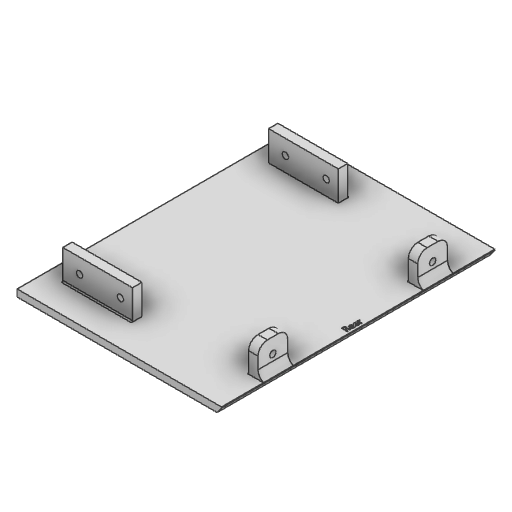
# Autodesk Inventor part: lowerSkidPlateRear
Saved by Autodesk Inventor 2025 (Build 290162000, 162)
## iProperties
Created: 2025-01-05
Part Number: lowerSkidPlateRear
Material: Generic
Document SubType Name: Modeling
Designer: derm
Density: 1 g/cm^3
Appearance: Default
Author: derm
Autodesk Inventor part; units mm, degrees
ref_plane "YZ Plane" through (0, 0, 0) normal (1, 0, 0) x (0, 1, 0)
ref_plane "XZ Plane" through (0, 0, 0) normal (0, 1, 0) x (-1, 0, 0)
ref_plane "XY Plane" through (0, 0, 0) normal (0, 0, 1) x (1, 0, 0)
sketch "Sketch1" plane through (0, 0, 0) normal (0, 1, 0) x (-1, 0, 0)
  line L0 (-87.5, 117) -> (87.5, 117)
  line L1 (87.5, 117) -> (87.5, -117)
  line L2 (87.5, -117) -> (-87.5, -117)
  line L3 (-87.5, -117) -> (-87.5, 117)
  line L4 (-87.5, 117) -> (87.5, -117) construction
  line L5 (87.5, 117) -> (-87.5, -117) construction
  point P0 (0, 0)
  dimension "d0" = 175
  dimension "d1" = 234
  constraints: 12 end point, 2 midpoint, 2 parallel, 1 horizontal, 1 perpendicular
  measures "d0" distance of L1.end L2.end
  measures "d1" distance of L0.end L1.end
extrude "Extrusion1" add sketch "Sketch1" along normal blind 6
sketch "Sketch2" plane through (0, 6, 0) normal (0, 1, 0) x (1, 0, 0)
  line L0 (87.5, 117) -> (-87.5, 117) projected
  line L1 (-87.5, 117) -> (-87.5, -117) projected
  line L2 (-87.5, -117) -> (87.5, -117) projected
  line L3 (87.5, -117) -> (87.5, 117) projected
  line L4 (76.2612, -82.1) -> (49.5135, -82.1)
  line L5 (74.806, 117.332) -> (74.806, -116.668)
  line L6 (49.5135, -82.1) -> (82.806, -82.1)
  line L7 (82.806, -82.1) -> (82.806, -55.7)
  line L8 (82.806, -55.7) -> (49.5135, -55.7)
  line L9 (49.5135, -55.7) -> (49.5135, -82.1)
  line L10 (82.806, -82.1) -> (49.5135, -82.1)
  line L11 (49.5135, -82.1) -> (49.5135, -81.1)
  line L12 (49.5135, -81.1) -> (82.806, -81.1)
  line L13 (82.806, -81.1) -> (82.806, -82.1)
  point P0 (0, 0)
  point P1 (74.806, -116.668)
  point P2 (66.1597, -55.7)
  point P3 (66.1597, -82.1)
  point P4 (74.806, -55.7)
  point P5 (70.1597, -82.1)
  point P6 (74.806, -81.1)
  dimension "d4" = 26.4
  dimension "d5" = 8
  dimension "d8" = 1
  constraints: 18 end point, 4 parallel, 2 horizontal, 2 midpoint, 2 perpendicular, 1 point on line, 3 other
  measures "d4" distance of point (66.16, -55.7) point (66.16, -82.1)
  measures "d8" distance between parallel lines of L12 L6
extrude "Extrusion2" add sketch "Sketch2" along normal blind 25.4 contours L5 L8 L7 L12
sketch "Sketch3" plane through (82.806, 6, 81.1) normal (1, 0, 0) x (0, 0, -1)
  line L0 (25.4, 0) -> (0, 0) projected
  line L1 (25.4, 0) -> (25.4, 25.4) projected
  line L2 (0, 25.4) -> (25.4, 25.4) projected
  line L3 (0, 0) -> (0, 25.4) projected
  circle A0 centre (12.7, 12.7) radius 2.75
  point P0 (81.1, -6)
  dimension "d9" = 5.5
  constraints: 1 centre point
  measures "d9" diameter of A0
extrude "Extrusion3" cut sketch "Sketch3" against normal blind 25.4 contours A0
fillet "Fillet1" radius 8 3 edges at (82.806, 6, 68.4) (78.806, 31.4, 55.7) (78.806, 31.4, 81.1)
sketch "Sketch4" plane through (0, 6, 0) normal (0, 1, 0) x (1, 0, 0)
  line L0 (87.5, -81.1) -> (74.806, -81.1) projected
  line L1 (74.806, -81.1) -> (74.806, -55.7) projected
  line L2 (74.806, -55.7) -> (87.5, -55.7) projected
  line L3 (87.5, 117) -> (-87.5, 117) projected
  line L4 (-87.5, 117) -> (-87.5, -117) projected
  line L5 (-87.5, -117) -> (87.5, -117) projected
  line L6 (87.5, -117) -> (87.5, -81.1) projected
  line L7 (-217.2403, -92.1) -> (36.7597, -92.1) projected
  line L8 (-7.3833, -87.6172) -> (32.2769, -47.957) projected
  line L9 (-13.6234, -92.1) -> (-73.3252, -92.1)
  line L10 (-73.3252, -92.1) -> (-73.3252, -84.1)
  line L11 (-73.3252, -84.1) -> (-13.6234, -84.1)
  line L12 (-13.6234, -84.1) -> (-13.6234, -92.1)
  line L13 (87.5, -55.7) -> (87.5, 117) projected
  point P0 (0, 0)
  point P1 (-73.3252, -92.1)
  dimension "d14" = 8
  constraints: 8 end point, 2 parallel, 1 horizontal, 1 perpendicular, 1 point on line, 1 vertical
  measures "d14" distance between parallel lines of L7 L11
extrude "Extrusion4" add sketch "Sketch4" along normal blind 25.4 contours L10 L11 L12 L7
sketch "Sketch5" plane through (-80, 6, 84.1) normal (0, 0, -1) x (-1, 0, 0)
  line L0 (-6.6748, 0) -> (-66.3766, 0) projected
  line L1 (-6.6748, 0) -> (-6.6748, 25.4) projected
  line L2 (-66.3766, 25.4) -> (-6.6748, 25.4) projected
  line L3 (-66.3766, 0) -> (-66.3766, 25.4) projected
  circle A0 centre (-56.0684, 12.7) radius 2.75
  circle A1 centre (-21.0684, 12.7) radius 2.75
  circle A2 centre (13.9316, 12.7) radius 2.75
  point P0 (-80, -6)
  dimension "d17" = 5.5
  dimension "d22" = 35
  constraints: 3 centre point, 1 horizontal, 4 other
  measures "d17" diameter of A0
  measures "d22" distance of A0.centre A1.centre
extrude "Extrusion5" cut sketch "Sketch5" against normal blind 25.4 contours A0 | A1 | A2
mirror "Mirror1" about plane through (0, 0, 0) normal (0, 0, 1) of "Extrusion2", "Extrusion3", "Fillet1", "Extrusion4", "Extrusion5"
sketch "Sketch8" plane through (87.5, 0, -117) normal (0, 0, -1) x (-1, 0, 0)
  line L0 (-8.2033, 16.4896) -> (-32.1539, 49.52) projected
  line L1 (0, 5.1764) -> (3.7534, 0)
  line L2 (0, 0) -> (175, 0) projected
  line L3 (175, 0) -> (175, 6) projected
  line L4 (0, 6) -> (175, 6) projected
  line L5 (0, 0) -> (0, 6) projected
  line L6 (0, 0) -> (0, 6) projected
  line L7 (0, 5.1764) -> (0, 0)
  line L8 (0, 0) -> (3.7534, 0)
  line L9 (175, 0) -> (0, 0) projected
  point P0 (87.5, 0)
  point P1 (3.7534, 0)
  constraints: 6 end point, 2 point on line, 1 collinear
extrude "Extrusion8" cut sketch "Sketch8" against normal through all contours L1 L2 L5
sketch "Sketch9" plane through (0, 6, 0) normal (0, 1, 0) x (1, 0, 0)
  line L0 (-13.6234, 84.1) -> (-73.3252, 84.1) projected
  line L1 (-73.3252, 84.1) -> (-73.3252, 92.1) projected
  line L2 (-73.3252, 92.1) -> (-13.6234, 92.1) projected
  line L3 (-13.6234, 92.1) -> (-13.6234, 84.1) projected
  line L4 (74.806, 81.1) -> (87.5, 81.1) projected
  line L5 (87.5, 81.1) -> (87.5, 117) projected
  line L6 (87.5, 117) -> (-87.5, 117) projected
  line L7 (-87.5, 117) -> (-87.5, -117) projected
  line L8 (-87.5, -117) -> (87.5, -117) projected
  line L9 (87.5, -117) -> (87.5, -81.1) projected
  line L10 (87.5, -81.1) -> (74.806, -81.1) projected
  line L11 (74.806, -81.1) -> (74.806, -55.7) projected
  line L12 (74.806, -55.7) -> (87.5, -55.7) projected
  line L13 (87.5, -55.7) -> (87.5, 55.7) projected
  line L14 (87.5, 55.7) -> (74.806, 55.7) projected
  line L15 (74.806, 55.7) -> (74.806, 81.1) projected
  line L16 (-73.3252, -84.1) -> (-13.6234, -84.1) projected
  line L17 (-13.6234, -84.1) -> (-13.6234, -92.1) projected
  line L18 (-13.6234, -92.1) -> (-73.3252, -92.1) projected
  line L19 (-73.3252, -92.1) -> (-73.3252, -84.1) projected
  line L20 (85.4318, -28.7814) -> (85.4318, 29.0837) construction
  line L21 (83.7466, 117) -> (83.7466, -117) projected
  spline S0 degree 2 poles (85.3323, -3.9151) (85.3607, -3.9151) (85.4081, -3.9388) (85.4413, -4.0147) (85.4556, -4.1569) (85.4556, -4.2708) knots 0 0 0 1 2 3 4 4 4
  spline S1 degree 2 poles (85.4556, -4.2708) (85.4556, -4.3751) (85.4413, -4.5031) (85.4034, -4.579) (85.3418, -4.6216) (85.2943, -4.6359) knots 0 0 0 1 2 3 4 4 4
  line L22 (85.2943, -4.6359) -> (84.1136, -5.1006)
  spline S2 degree 2 poles (84.1136, -5.1006) (83.9097, -5.1812) (83.5731, -5.3566) (83.3312, -5.5985) (83.1937, -5.9209) (83.1937, -6.1532) knots 0 0 0 1 2 3 4 4 4
  line L23 (83.1937, -6.1532) -> (83.1937, -6.599)
  line L24 (83.1937, -6.599) -> (85.3323, -6.599)
  spline S3 degree 2 poles (85.3323, -6.599) (85.3607, -6.599) (85.4081, -6.6322) (85.4366, -6.708) (85.4556, -6.8361) (85.4556, -6.9309) knots 0 0 0 1 2 3 4 4 4
  spline S4 degree 2 poles (85.4556, -6.9309) (85.4556, -7.0305) (85.4366, -7.1585) (85.4081, -7.2344) (85.3607, -7.2676) (85.3323, -7.2676) knots 0 0 0 1 2 3 4 4 4
  line L25 (85.3323, -7.2676) -> (80.6758, -7.2676)
  spline S5 degree 2 poles (80.6758, -7.2676) (80.5241, -7.2676) (80.4056, -7.1063) (80.4056, -7.021) knots 0 0 0 1 2 2 2
  line L26 (80.4056, -7.021) -> (80.4056, -5.9493)
  spline S6 degree 2 poles (80.4056, -5.9493) (80.4056, -5.7597) (80.4245, -5.5084) (80.4387, -5.4088) knots 0 0 0 1 2 2 2
  spline S7 degree 2 poles (80.4387, -5.4088) (80.4862, -5.1148) (80.7043, -4.6691) (81.041, -4.3656) (81.4725, -4.2138) (81.7333, -4.2138) knots 0 0 0 1 2 3 4 4 4
  spline S8 degree 2 poles (81.7333, -4.2138) (81.9846, -4.2138) (82.3829, -4.3514) (82.6911, -4.6074) (82.9187, -4.9631) (82.9946, -5.1859) knots 0 0 0 1 2 3 4 4 4
  spline S9 degree 2 poles (82.9946, -5.1859) (83.0515, -5.0626) (83.2174, -4.8587) (83.4498, -4.6833) (83.7533, -4.5268) (83.9429, -4.4509) knots 0 0 0 1 2 3 4 4 4
  line L27 (83.9429, -4.4509) -> (85.0478, -4.0005)
  spline S10 degree 2 poles (85.0478, -4.0005) (85.19, -3.9436) (85.2991, -3.9151) (85.3323, -3.9151) knots 0 0 0 1 2 2 2
  spline S11 degree 2 poles (81.7996, -4.9204) (81.5056, -4.9204) (81.0979, -5.1859) (81.0078, -5.4941) knots 0 0 0 1 2 2 2
  spline S12 degree 2 poles (81.0078, -5.4941) (80.9793, -5.5937) (80.9556, -5.8355) (80.9556, -6.0347) knots 0 0 0 1 2 2 2
  line L28 (80.9556, -6.0347) -> (80.9556, -6.599)
  line L29 (80.9556, -6.599) -> (82.6532, -6.599)
  line L30 (82.6532, -6.599) -> (82.6532, -5.9446)
  spline S13 degree 2 poles (82.6532, -5.9446) (82.6532, -5.6838) (82.5251, -5.295) (82.2928, -5.0389) (81.9846, -4.9204) (81.7996, -4.9204) knots 0 0 0 1 2 3 4 4 4
  spline S14 degree 2 poles (83.4356, -0.0411) (83.5873, -0.0411) (83.7153, -0.1928) (83.7153, -0.2924) knots 0 0 0 1 2 2 2
  line L31 (83.7153, -0.2924) -> (83.7153, -2.5922)
  spline S15 degree 2 poles (83.7153, -2.5922) (84.0046, -2.5922) (84.474, -2.4736) (84.8059, -2.2033) (84.9861, -1.7671) (84.9861, -1.4494) knots 0 0 0 1 2 3 4 4 4
  spline S16 degree 2 poles (84.9861, -1.4494) (84.9861, -1.1981) (84.9055, -0.8092) (84.8012, -0.5247) (84.7206, -0.3398) (84.7206, -0.2924) knots 0 0 0 1 2 3 4 4 4
  spline S17 degree 2 poles (84.7206, -0.2924) (84.7206, -0.2639) (84.749, -0.2213) (84.8012, -0.1976) (84.9008, -0.1881) (84.9719, -0.1881) knots 0 0 0 1 2 3 4 4 4
  spline S18 degree 2 poles (84.9719, -0.1881) (85.0193, -0.1881) (85.0952, -0.1976) (85.1521, -0.207) (85.1995, -0.2355) (85.2422, -0.2782) (85.3418, -0.4868) (85.4318, -0.8187) (85.5077, -1.2597) (85.5077, -1.5063) knots 0 0 0 1 2 3 4 5 6 7 8 8 8
  spline S19 degree 2 poles (85.5077, -1.5063) (85.5077, -1.9378) (85.2659, -2.5874) (84.7917, -3.0284) (84.0757, -3.256) (83.6015, -3.256) knots 0 0 0 1 2 3 4 4 4
  spline S20 degree 2 poles (83.6015, -3.256) (83.151, -3.256) (82.4303, -3.0237) (81.9324, -2.5827) (81.6621, -1.9615) (81.6621, -1.5774) knots 0 0 0 1 2 3 4 4 4
  spline S21 degree 2 poles (81.6621, -1.5774) (81.6621, -1.1649) (81.9277, -0.5864) (82.3734, -0.2165) (82.9756, -0.0411) (83.317, -0.0411) knots 0 0 0 1 2 3 4 4 4
  line L32 (83.317, -0.0411) -> (83.4356, -0.0411)
  spline S22 degree 2 poles (83.2459, -0.686) (82.7385, -0.6765) (82.1648, -1.1459) (82.1648, -1.6106) knots 0 0 0 1 2 2 2
  spline S23 degree 2 poles (82.1648, -1.6106) (82.1648, -1.8477) (82.3449, -2.2081) (82.6389, -2.4499) (83.0325, -2.5827) (83.2459, -2.5922) knots 0 0 0 1 2 3 4 4 4
  line L33 (83.2459, -2.5922) -> (83.2459, -0.686)
  spline S24 degree 2 poles (85.337, 3.5674) (85.3844, 3.5674) (85.4318, 3.5058) (85.4556, 3.3967) (85.4556, 3.2924) knots 0 0 0 1 2 3 3 3
  spline S25 degree 2 poles (85.4556, 3.2924) (85.4556, 3.1928) (85.4318, 3.0695) (85.3844, 3.0174) (85.337, 3.0174) knots 0 0 0 1 2 3 3 3
  line L34 (85.337, 3.0174) -> (84.9909, 3.0174)
  spline S26 degree 2 poles (84.9909, 3.0174) (85.2327, 2.7898) (85.5077, 2.2255) (85.5077, 1.9125) knots 0 0 0 1 2 2 2
  spline S27 degree 2 poles (85.5077, 1.9125) (85.5077, 1.6328) (85.3655, 1.187) (85.0904, 0.8741) (84.6921, 0.6986) (84.4408, 0.6986) knots 0 0 0 1 2 3 4 4 4
  spline S28 degree 2 poles (84.4408, 0.6986) (84.1421, 0.6986) (83.7058, 0.9405) (83.4166, 1.3909) (83.2743, 2.0406) (83.2743, 2.4484) knots 0 0 0 1 2 3 4 4 4
  line L35 (83.2743, 2.4484) -> (83.2743, 2.932)
  line L36 (83.2743, 2.932) -> (83.0041, 2.932)
  spline S29 degree 2 poles (83.0041, 2.932) (82.8002, 2.932) (82.4919, 2.8467) (82.288, 2.657) (82.1837, 2.3535) (82.1837, 2.1307) knots 0 0 0 1 2 3 4 4 4
  spline S30 degree 2 poles (82.1837, 2.1307) (82.1837, 1.8936) (82.2975, 1.519) (82.4303, 1.2345) (82.5441, 1.0448) (82.5441, 0.9974) knots 0 0 0 1 2 3 4 4 4
  spline S31 degree 2 poles (82.5441, 0.9974) (82.5441, 0.9642) (82.5109, 0.9215) (82.4493, 0.8836) (82.3544, 0.8693) (82.2975, 0.8693) knots 0 0 0 1 2 3 4 4 4
  spline S32 degree 2 poles (82.2975, 0.8693) (82.1979, 0.8693) (82.0841, 0.8978) (81.9846, 1.0021) (81.8471, 1.2582) (81.738, 1.5901) (81.6621, 1.9884) (81.6621, 2.1876) knots 0 0 0 1 2 3 4 5 6 6 6
  spline S33 degree 2 poles (81.6621, 2.1876) (81.6621, 2.5669) (81.8328, 3.0932) (82.1648, 3.4204) (82.6532, 3.5674) (82.9803, 3.5674) knots 0 0 0 1 2 3 4 4 4
  line L37 (82.9803, 3.5674) -> (85.337, 3.5674)
  line L38 (83.739, 2.932) -> (83.739, 2.382)
  spline S34 degree 2 poles (83.739, 2.382) (83.739, 2.1212) (83.8291, 1.7323) (84.0046, 1.4715) (84.2511, 1.353) (84.4076, 1.353) knots 0 0 0 1 2 3 4 4 4
  spline S35 degree 2 poles (84.4076, 1.353) (84.6826, 1.353) (85.0051, 1.6992) (85.0051, 2.0121) knots 0 0 0 1 2 2 2
  spline S36 degree 2 poles (85.0051, 2.0121) (85.0051, 2.2634) (84.749, 2.6949) (84.4835, 2.932) knots 0 0 0 1 2 2 2
  line L39 (84.4835, 2.932) -> (83.739, 2.932)
  spline S37 degree 2 poles (82.0652, 6.7918) (82.1505, 6.7918) (82.2691, 6.7823) (82.3355, 6.7586) (82.3687, 6.7254) (82.3687, 6.697) knots 0 0 0 1 2 3 4 4 4
  spline S38 degree 2 poles (82.3687, 6.697) (82.3687, 6.6638) (82.3355, 6.5737) (82.3023, 6.4599) (82.2691, 6.3224) (82.2691, 6.2418) knots 0 0 0 1 2 3 4 4 4
  spline S39 degree 2 poles (82.2691, 6.2418) (82.2691, 6.1422) (82.3449, 5.9573) (82.5251, 5.7486) (82.8239, 5.5258) (83.0372, 5.3883) knots 0 0 0 1 2 3 4 4 4
  line L40 (83.0372, 5.3883) -> (85.337, 5.3883)
  spline S40 degree 2 poles (85.337, 5.3883) (85.3655, 5.3883) (85.4081, 5.3551) (85.4413, 5.2887) (85.4556, 5.1654) (85.4556, 5.0658) knots 0 0 0 1 2 3 4 4 4
  spline S41 degree 2 poles (85.4556, 5.0658) (85.4556, 4.971) (85.4413, 4.8477) (85.4081, 4.7766) (85.3655, 4.7481) (85.337, 4.7481) knots 0 0 0 1 2 3 4 4 4
  line L41 (85.337, 4.7481) -> (81.8376, 4.7481)
  spline S42 degree 2 poles (81.8376, 4.7481) (81.8091, 4.7481) (81.7664, 4.7718) (81.7285, 4.843) (81.719, 4.952) (81.719, 5.0374) knots 0 0 0 1 2 3 4 4 4
  spline S43 degree 2 poles (81.719, 5.0374) (81.719, 5.1227) (81.7285, 5.2365) (81.7664, 5.2982) (81.8091, 5.3266) (81.8376, 5.3266) knots 0 0 0 1 2 3 4 4 4
  line L42 (81.8376, 5.3266) -> (82.3497, 5.3266)
  spline S44 degree 2 poles (82.3497, 5.3266) (82.1363, 5.4689) (81.8708, 5.7249) (81.719, 5.9478) (81.6621, 6.1707) (81.6621, 6.2845) knots 0 0 0 1 2 3 4 4 4
  spline S45 degree 2 poles (81.6621, 6.2845) (81.6621, 6.3319) (81.6716, 6.4599) (81.7048, 6.6022) (81.7427, 6.716) (81.7807, 6.7586) (81.8186, 6.7776) (81.8708, 6.7871) (81.9751, 6.7918) (82.0652, 6.7918) knots 0 0 0 1 2 3 4 5 6 7 8 8 8
  point P0 (0, 0)
  constraints: 2 end point, 1 parallel, 1 vertical
extrude "Extrusion9" cut sketch "Sketch9" against normal blind 0.4 contours L40 S40 S41 L41 L21 | L21 L41 S42 S43 L42 S44 S45 S37 S38 S39 L40 | L37 S24 S25 L34 S26 S27 S28 L21 S34 S35 S36 L39 | L21 L39 L38 S34 S28 L35 L36 S29 S30 S31 S32 S33 L37 | L25 S5 L26 S6 S7 S8 S9 L21 S2 L23 L24 | L21 L24 S3 S4 L25 | L21 S9 L27 S10 S0 S1 L22 S2 | S15 S16 S17 S18 S19 L21 | L21 S19 S20 S21 L32 S14 L31 S15
fillet "Fillet2" radius 1 4 edges at (-43.4743, 6, 92.1) (-43.4743, 6, -92.1) (74.806, 6, 68.4) (74.806, 6, -68.4)
sketch "Sketch6" plane through (0, 6, 0) normal (0, 1, 0) x (1, 0, 0)
  line L0 (-13.6234, 84.1) -> (-73.3252, 84.1) projected
  line L1 (-73.3252, 84.1) -> (-73.3252, 92.1) projected
  line L2 (-73.3252, 92.1) -> (-13.6234, 92.1) projected
  line L3 (-13.6234, 92.1) -> (-13.6234, 84.1) projected
  line L4 (78.1597, 55.7) -> (62.1597, 55.7) projected
  line L5 (62.1597, 55.7) -> (62.1597, 81.1) projected
  line L6 (62.1597, 81.1) -> (78.1597, 81.1) projected
  line L7 (78.1597, 55.7) -> (78.1597, 81.1) projected
  line L8 (-73.3252, -84.1) -> (-13.6234, -84.1) projected
  line L9 (-13.6234, -84.1) -> (-13.6234, -92.1) projected
  line L10 (-13.6234, -92.1) -> (-73.3252, -92.1) projected
  line L11 (-73.3252, -92.1) -> (-73.3252, -84.1) projected
  line L12 (78.1597, -81.1) -> (62.1597, -81.1) projected
  line L13 (62.1597, -81.1) -> (62.1597, -55.7) projected
  line L14 (62.1597, -55.7) -> (78.1597, -55.7) projected
  line L15 (78.1597, -81.1) -> (78.1597, -55.7) projected
  line L16 (87.5, 117) -> (-80, 117) projected
  line L17 (-80, 117) -> (-80, -117) projected
  line L18 (-80, -117) -> (87.5, -117) projected
  line L19 (80, -117) -> (80, 117) projected
  line L20 (-14.0403, 77.5) -> (-69.0403, 77.5)
  line L21 (-69.0403, 77.5) -> (-69.0403, -77.5)
  line L22 (-69.0403, -77.5) -> (-14.0403, -77.5)
  line L23 (-14.0403, -77.5) -> (-14.0403, 77.5)
  line L24 (-14.0403, 77.5) -> (-69.0403, -77.5) construction
  line L25 (-69.0403, 77.5) -> (-14.0403, -77.5) construction
  line L26 (87.5, -117) -> (87.5, 117) projected
  line L27 (80, 0) -> (-80, 0)
  line L28 (-9.0403, -82.5) -> (-74.0403, -82.5)
  line L29 (-74.0403, -82.5) -> (-74.0403, 82.5)
  line L30 (-74.0403, 82.5) -> (-9.0403, 82.5)
  line L31 (-9.0403, 82.5) -> (-9.0403, -82.5)
  point P0 (0, 0)
  point P1 (-41.5403, 0)
  dimension "d27" = 155
  dimension "d28" = 55
  dimension "d29" = 76.2
  dimension "d30" = 5
  constraints: 22 end point, 4 parallel, 3 midpoint, 2 perpendicular, 1 horizontal, 1 point on line, 5 other
  measures "d27" distance of L22.end L20.start
  measures "d28" distance of L21.end L22.end
  measures "d29" distance between parallel lines of L5 L23
  measures "d30" distance between parallel lines of L31 L23
sketch "Sketch7" plane through (0, 6, 0) normal (0, 1, 0) x (1, 0, 0)
  line L0 (-14.0403, 77.5) -> (-69.0403, 77.5) projected
  line L1 (-69.0403, 77.5) -> (-69.0403, -77.5) projected
  line L2 (-69.0403, -77.5) -> (-14.0403, -77.5) projected
  line L3 (-14.0403, -77.5) -> (-14.0403, 77.5) projected
  point P0 (0, 0)
body "Solid1"
